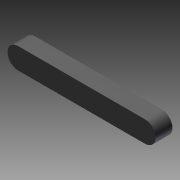
# Autodesk Inventor part: K0696.110X70
Saved by Autodesk Inventor 2011 SP1 (Build 150282100, 282)
## iProperties
Created: 2018-03-23
Part Number: K0696.110X70
Catalog Web Link: www.cadenas.de
Description: K0696-Parallel keys DIN 6885 A
Vendor: KIPP
Document SubType Name: Modeling
Designer: psAdmin
Manufacturer: KIPP
Mass: 5.42832 g
Surface Area: 25.6841 cm^2
Volume: 5.42832 cm^3
Density: 1 g/cm^3
Category: PARTsolutions
Company: KIPP
Title: K0696.110X70
Author: Cadenas PARTsolutions
Comments: Parallel keys DIN 6885 A
PSOL_IDENT_0: {$CADENAS_DATA\23d-libs\kipp\data\03000\03288.prj},169 {VTYP=3D},{NB=K0696.110X70},{LINA=K0696.110X7
PSOL_IDENT_1: 0},{NN=K0696},{DATE=19.03.2018 11:02:13},{GEOMDATE=19.03.2018 07:25:30},{VERSION=v1},{LINEID=4370},{
PSOL_IDENT_2: LINESUBID=-1},{WBVAR=}  {NB=K0696.110X70},{LINA=K0696.110X70},{KT=X},{BESTKIPP=K0696.110X70},{BEST=0
PSOL_IDENT_3: 3288-110X70},{AUSF=Edelstahl},{B=10},{H=8},{L=70},{BS=Infotext},{FILTER=KIPP,NORELEM},{LZR=0}
NN: K0696
NT: Parallel keys DIN 6885 A
NB: K0696.110X70
NBSYN: $BESTKIPP.
LINA: K0696.110X70
BESTKIPP: K0696.110X70
AUSF: stainless steel
B: 10
H: 8
L: 70
BS: Infotext
SUPPLIER: KIPP
ARTICLENO: K0696.110X70
BOMINFO: K0696.110X70
CREATOR: CADENAS GmbH
Autodesk Inventor part; units mm, degrees
sketch "Sketch_1" plane through (0, 0, 0) normal (0, 1, 0) x (-1, 0, 0)
  arc A0 (35, 0) -> (30, 5) centre (30, 0) ccw
  line L0 (30, 5) -> (-30, 5)
  arc A1 (-30, 5) -> (-35, 0) centre (-30, 0) ccw
  arc A2 (-35, 0) -> (-30, -5) centre (-30, 0) ccw
  line L1 (-30, -5) -> (30, -5)
  arc A3 (30, -5) -> (35, 0) centre (30, 0) ccw
  constraints: 8 point on circle, 4 centre point, 4 end point
extrude "Extrusion1" add sketch "Sketch_1" along normal mid plane 8
ref_plane "bp_b_oben_XY" through (30, 0, -5) normal (0, 1, 0) x (1, 0, 0)
ref_plane "bp_b_oben_YZ" through (30, 0, -5) normal (1, 0, 0) x (0, 0, -1)
ref_plane "bp_b_oben_ZX" through (30, 0, -5) normal (0, 0, -1) x (0, 1, 0)
ref_plane "bp_b_unten_XY" through (30, 0, 5) normal (0, 1, 0) x (1, 0, 0)
ref_plane "bp_b_unten_YZ" through (30, 0, 5) normal (1, 0, 0) x (0, 0, -1)
ref_plane "bp_b_unten_ZX" through (30, 0, 5) normal (0, 0, -1) x (0, 1, 0)
ref_plane "bp_h_oben_XY" through (0, 4, 0) normal (0, 0, 1) x (1, 0, 0)
ref_plane "bp_h_oben_YZ" through (0, 4, 0) normal (1, 0, 0) x (0, 1, 0)
ref_plane "bp_h_oben_ZX" through (0, 4, 0) normal (0, 1, 0) x (0, 0, 1)
ref_plane "bp_h_unten_XY" through (0, -4, 0) normal (0, 0, 1) x (1, 0, 0)
ref_plane "bp_h_unten_YZ" through (0, -4, 0) normal (1, 0, 0) x (0, 1, 0)
ref_plane "bp_h_unten_ZX" through (0, -4, 0) normal (0, 1, 0) x (0, 0, 1)
ref_plane "bp_l_links_XY" through (-35, 0, 0) normal (0, 1, 0) x (1, 0, 0)
ref_plane "bp_l_links_YZ" through (-35, 0, 0) normal (1, 0, 0) x (0, 0, -1)
ref_plane "bp_l_links_ZX" through (-35, 0, 0) normal (0, 0, -1) x (0, 1, 0)
ref_plane "bp_l_rechts_XY" through (35, 0, 0) normal (0, 1, 0) x (1, 0, 0)
ref_plane "bp_l_rechts_YZ" through (35, 0, 0) normal (1, 0, 0) x (0, 0, -1)
ref_plane "bp_l_rechts_ZX" through (35, 0, 0) normal (0, 0, -1) x (0, 1, 0)
body "Solid1"
